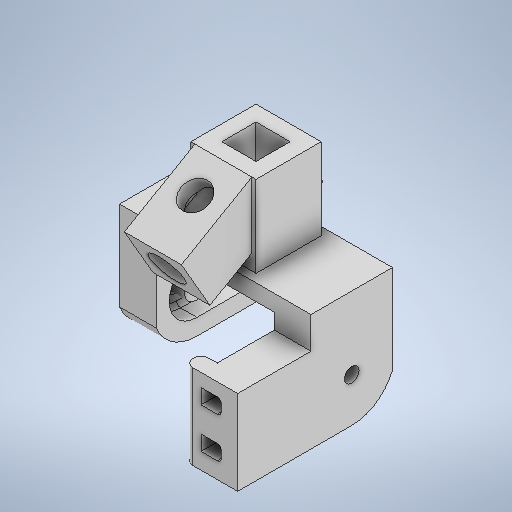
# Autodesk Inventor part: øvre del av kne Andre versjon
Saved by Autodesk Inventor 2025.1 (Build 291241020, 241B)
## iProperties
Created: 2024-10-04
Part Number: øvre del av kne Andre versjon
Material: Generic
Document SubType Name: Modeling
Designer: morte
Density: 1 g/cm^3
Appearance: Default
Author: morte
Autodesk Inventor part; units mm, degrees
ref_plane "XZ Plane" through (0, 0, 0) normal (0, 1, 0) x (-1, 0, 0)
ref_plane "XY Plane" through (0, 0, 0) normal (0, 0, 1) x (1, 0, 0)
sketch "Sketch1" plane through (0, 0, 0) normal (0, 0, 1) x (1, 0, 0)
  line L0 (0, 0) -> (0, 12.3)
  line L1 (0, 12.3) -> (14.5, 12.3)
  line L2 (14.5, 12.3) -> (14.5, 0)
  line L3 (14.5, 0) -> (19, 0)
  line L4 (19, 0) -> (19, 14.3)
  line L5 (19, 14.3) -> (-4.5, 14.3)
  line L6 (-4.5, 14.3) -> (-4.5, 0)
  line L7 (-4.5, 0) -> (0, 0)
  dimension "d6" = 12.3
  dimension "d7" = 14.5
  dimension "d8" = 4.5
  dimension "d9" = 14.3
  dimension "d10" = 23.5
  dimension "d108" = 12.3
  dimension "d205" = 4.5
  constraints: 16 end point, 3 perpendicular, 3 vertical, 2 horizontal
  measures "d6" distance of L0.start L0.end
  measures "d7" distance of L0.end L1.end
  measures "d8" distance of L2.end L3.end
  measures "d9" distance of L3.end L4.end
  measures "d10" distance of L4.end L5.end
  measures "d108" distance of L1.end L2.end
  measures "d205" distance of L6.end L0.start
extrude "Extrusion1" add sketch "Sketch1" along normal mid plane 10
sketch "Sketch2" plane through (-4.5, 14.3, 5) normal (0, 1, 0) x (1, 0, 0)
  line L0 (0, 10) -> (0, 0) projected
  line L1 (0, 10) -> (23.5, 10) projected
  line L2 (0, 0) -> (23.5, 10)
  line L3 (23.5, 0) -> (0, 0) projected
  line L4 (0, 10) -> (23.5, 0)
  line L5 (9.65, 2.9) -> (13.85, 2.9)
  line L6 (13.85, 2.9) -> (13.85, 7.1)
  line L7 (13.85, 7.1) -> (9.65, 7.1)
  line L8 (9.65, 7.1) -> (9.65, 2.9)
  line L9 (9.65, 2.9) -> (13.85, 7.1) construction
  line L10 (13.85, 2.9) -> (9.65, 7.1) construction
  line L11 (7.75, 1) -> (15.75, 1)
  line L12 (15.75, 1) -> (15.75, 9)
  line L13 (15.75, 9) -> (7.75, 9)
  line L14 (7.75, 9) -> (7.75, 1)
  line L15 (7.75, 1) -> (15.75, 9) construction
  line L16 (15.75, 1) -> (7.75, 9) construction
  point P0 (4.5, 5)
  point P1 (11.75, 5)
  dimension "d11" = 4.2
  dimension "d12" = 4.2
  dimension "d13" = 8
  dimension "d14" = 8
  constraints: 28 end point, 5 midpoint, 4 parallel, 2 horizontal, 2 perpendicular, 1 point on line
  measures "d11" distance of L6.end L7.end
  measures "d12" distance of L5.end L6.end
  measures "d13" distance of L12.end L13.end
  measures "d14" distance of L11.end L12.end
extrude "Extrusion2" add sketch "Sketch2" along normal blind 10 contours L14 L13 L12 L2 L6 L7 L8 L4 | L4 L8 L2 L14 | L2 L8 L5 L6 L4 L12 L11 L14 | L12 L4 L6 L2
sketch "Sketch3" plane through (0, 0, 5) normal (1, 0, 0) x (0, 0, -1)
  line L0 (10, 0) -> (0, 0) projected
  line L1 (0, 0) -> (5, 0)
  line L2 (10, 14.3) -> (0, 14.3) projected
  line L3 (6.95, 14.3) -> (3.05, 14.3)
  line L4 (5, 0) -> (5, 2)
  line L5 (8.4, 5.4) -> (17.767, 5.4) construction
  line L6 (6.8, 5.4) -> (16.167, 5.4) construction
  line L7 (1.6, 5.4) -> (10.967, 5.4) construction
  line L8 (3.2, 5.4) -> (12.567, 5.4) construction
  line L9 (5, 5.4) -> (5, 0)
  line L10 (5, 8.8) -> (5, 10.4)
  line L11 (5, 10.4) -> (19, 10.4)
  line L12 (5, 0) -> (19, 0)
  line L13 (19, 0) -> (19, 10.4)
  line L14 (5, 8.8) -> (5, 0)
  point P0 (1.9, 14.3)
  point P1 (8.1, 14.3)
  point P2 (10, 0)
  dimension "d17" = 5
  dimension "d111" = 2
  dimension "d172" = 1.6
  dimension "d173" = 14
  dimension "d174" = 14
  constraints: 26 end point, 6 point on line, 4 horizontal, 2 collinear, 2 perpendicular, 2 vertical, 1 midpoint
  measures "d17" distance of L0.end L1.end
  measures "d111" distance of L1.end L4.end
  measures "d172" distance of L10.start L10.end
  measures "d173" distance of L10.end L11.end
  measures "d174" distance of L12.start L12.end
extrude "Extrusion3" add sketch "Sketch3" against normal blind 4.5
ref_plane "Work Plane1" through (10.75, 0, 0) normal (1, 0, 0) x (0, 1, 0)
sketch "Sketch15" plane through (10.75, 0, 0) normal (1, 0, 0) x (0, 1, 0)
  line L0 (24.3, -4) -> (24.3, 4) projected
  line L1 (24.3, 4) -> (19.3, 12.6603)
  line L2 (24.3, 4) -> (34.3, 4) construction
  line L3 (24.3, 4) -> (16.3, 4)
  line L4 (14.3, 4) -> (24.3, 4) projected
  line L5 (19.3, 12.6603) -> (13.2378, 9.1603)
  line L6 (13.2378, 9.1603) -> (16.2171, 4)
  line L7 (13.2378, 9.1603) -> (19.1964, 9.1603) construction
  point P0 (0, 0)
  point P1 (18.5265, 4)
  dimension "d83" = 10
  dimension "d84" = 120
  dimension "d85" = 8
  dimension "d93" = 7
  dimension "d94" = 60
  constraints: 12 end point, 2 equal length, 2 horizontal, 2 point on line
  measures "d83" distance of L0.end L1.end
  measures "d84" angle of L2 L1
  measures "d85" distance of L0.end L3.end
  measures "d93" distance of L1.end L5.end
  measures "d94" angle of L6 L7
extrude "Extrusion13" add sketch "Sketch15" against normal blind 7
sketch "Sketch17" plane through (3.75, 19.3, 12.6603) normal (0, -0.5, 0.866) x (1, 0, 0)
  line L0 (7, -7) -> (0, -7) projected
  line L1 (0, 0) -> (3.5, 0)
  line L2 (3.5, 0) -> (3.5, -3.5)
  circle A0 centre (3.5, -3.5) radius 2.1
  point P0 (-3.75, -23.0444)
  point P1 (0.25, -7)
  point P2 (6.5, -7)
  dimension "d119" = 3.5
  dimension "d120" = 3.5
  dimension "d121" = 4.2
  constraints: 4 end point, 1 centre point, 1 coincident, 1 horizontal, 1 perpendicular
  measures "d119" distance of L1.start L1.end
  measures "d120" distance of L1.end L2.end
  measures "d121" diameter of A0
extrude "Extrusion15" cut sketch "Sketch17" against normal blind 13
sketch "Sketch22" plane through (14.5, 0, 5) normal (-1, 0, 0) x (0, 0, 1)
  line L0 (-10, 0) -> (0, 0) projected
  line L1 (0, 0) -> (-5, 0)
  line L2 (-5, 0) -> (0.4, 0) construction
  line L3 (9, 8.8) -> (9, 0)
  line L4 (9, 0) -> (-5, 0)
  line L5 (9, 9.4295) -> (9, 0)
  line L6 (-5, 10.4) -> (9, 10.4)
  line L7 (9, 10.4) -> (9, 9.4295)
  line L8 (-5, 10.4) -> (-5, 0)
  point P0 (0, 0)
  constraints: 16 end point, 4 collinear, 1 horizontal, 1 perpendicular
extrude "Extrusion20" add sketch "Sketch22" against normal blind 4.5
sketch "Sketch23" plane through (14.5, 0, -5) normal (-1, 0, 0) x (0, 0, 1)
  line L0 (0, 14.3) -> (0, 0) projected
  line L1 (0, 0) -> (5, 0)
  line L2 (0, 0) -> (19, 0) projected
  line L3 (5, 0) -> (5, 5.4)
  circle A0 centre (5, 5.4) radius 1.55
  circle A1 centre (5, 5.4) radius 3.4
  line L4 (5, 2) -> (20, 2)
  line L5 (5, 3.85) -> (20, 3.85)
  line L6 (5, 6.95) -> (20, 6.95)
  line L7 (5, 8.8) -> (20, 8.8)
  line L8 (20, 8.8) -> (20, 6.95)
  line L9 (20, 3.85) -> (20, 2)
  point P0 (8.0261, 3.85)
  point P1 (8.0261, 6.95)
  dimension "d161" = 5.4
  dimension "d162" = 3.1
  dimension "d163" = 6.8
  dimension "d164" = 15
  dimension "d165" = 15
  dimension "d166" = 15
  constraints: 16 end point, 4 point on circle, 4 tangent, 3 perpendicular, 2 centre point, 2 coincident, 2 horizontal, 2 point on line, 1 collinear, 1 vertical
  measures "d161" distance of L1.end L3.end
  measures "d162" diameter of A0
  measures "d163" diameter of A1
  measures "d164" distance of L4.start L4.end
  measures "d165" distance of L5.start L5.end
  measures "d166" distance of L6.start L6.end
extrude "Extrusion21" cut sketch "Sketch23" against normal blind 2.5 contours A1 L6 A0 L3 | L3 L5 A1 | A1 L5 L9 L4 | A0 L6 A1 L5 | L7 L8 L6 A1
sketch "Sketch24" plane through (14.5, 5.4, 0) normal (-1, 0, 0) x (0, 0, 1)
  circle A0 centre (0, 0) radius 0.9
  point P0 (0, -5.4)
  dimension "d169" = 1.8
  constraints: 1 centre point
  measures "d169" diameter of A0
extrude "Extrusion22" cut sketch "Sketch24" against normal through all
sketch "Sketch25" plane through (0, 0, 5) normal (1, 0, 0) x (0, 0, -1)
  line L0 (19, 0) -> (0, 0) projected
  line L1 (0, 0) -> (5, 0)
  line L2 (5, 0) -> (5, 5.4)
  line L3 (5, 0) -> (10.4, 0) construction
  circle A0 centre (5, 5.4) radius 1.55
  circle A1 centre (5, 5.4) radius 3.4
  line L4 (5, 8.8) -> (20, 8.8)
  line L5 (5, 6.95) -> (20, 6.95)
  line L6 (5, 3.85) -> (20, 3.85)
  line L7 (5, 2) -> (20, 2)
  line L8 (20, 2) -> (20, 3.85)
  line L9 (20, 6.95) -> (20, 8.8)
  point P0 (8.0261, 6.95)
  point P1 (8.0261, 3.85)
  dimension "d175" = 5.4
  dimension "d176" = 90
  dimension "d177" = 3.1
  dimension "d178" = 6.8
  dimension "d179" = 15
  dimension "d180" = 15
  dimension "d181" = 15
  dimension "d182" = 15
  constraints: 18 end point, 4 horizontal, 4 perpendicular, 4 point on circle, 4 tangent, 2 centre point, 2 coincident, 2 point on line
  measures "d175" distance of L1.end L2.end
  measures "d176" angle of L3 L2
  measures "d177" diameter of A0
  measures "d178" diameter of A1
  measures "d179" distance of L4.start L4.end
  measures "d180" distance of L5.start L5.end
  measures "d181" distance of L6.start L6.end
  measures "d182" distance of L7.start L7.end
extrude "Extrusion23" cut sketch "Sketch25" against normal blind 2.5 contours A1 L5 A0 L2 | L2 L6 A1 | A1 L6 L8 L7 | A0 L5 A1 L6 | L4 L9 L5 A1
sketch "Sketch26" plane through (0, 5.4, 0) normal (1, 0, 0) x (0, 0, -1)
  circle A0 centre (0, 0) radius 0.9
  point P0 (0, -5.4)
  dimension "d185" = 1.8
  constraints: 1 centre point
  measures "d185" diameter of A0
extrude "Extrusion24" cut sketch "Sketch26" against normal through all
sketch "Sketch27" plane through (0, 5.4, 0) normal (1, 0, 0) x (0, 0, -1)
  circle A0 centre (0, 0) radius 0.9 projected
  arc A1 (-5, -2.0396) -> (0, -5.4) centre (0, 0) ccw
  line L0 (-5, 8.9) -> (-5, -5.4) projected
  line L1 (-5, -2.0396) -> (-5, -5.4)
  line L2 (-5, -5.4) -> (0, -5.4)
  constraints: 4 end point, 3 point on circle, 2 point on line, 1 centre point, 1 coincident, 1 collinear, 1 perpendicular
extrude "Extrusion25" cut sketch "Sketch27" against normal through all contours A1 L2 L0
sketch "Sketch28" plane through (14.5, 5.4, 0) normal (-1, 0, 0) x (0, 0, 1)
  arc A0 (-5, -2.0388) -> (0.0007, -5.4) centre (0.0003, 0) ccw
  line L0 (-5, 8.9) -> (-5, -5.4) projected
  line L1 (-5, -2.0388) -> (-5, -5.4)
  line L2 (-5, -5.4) -> (0, -5.4)
  constraints: 4 end point, 3 point on circle, 2 point on line, 1 centre point, 1 collinear, 1 perpendicular
extrude "Extrusion26" cut sketch "Sketch28" against normal through all
fillet "Fillet9" radius 0.5 12 edges at (17, 8.8, 7) (17, 2, 7) (17, 5.4, -3.4) (17, 5.4, -1.55) (17, 6.95, 8.5131) (17, 3.85, 8.5131) (-2.5, 8.8, -7) (-2.5, 2, -7) (-2.5, 5.4, 3.4) (-2.5, 6.95, -8.5131) (-2.5, 3.85, -8.5131) (-2.5, 5.4, 1.55)
sketch "Sketch29" plane through (0, 3.85, -14) normal (1, 0, 0) x (0, 0, -1)
  line L0 (0, 6.55) -> (0, -3.85) projected
  line L1 (0, -3.85) -> (-2, -3.85)
  line L2 (0, -3.85) -> (-14, -3.85) projected
  line L3 (-2, -3.85) -> (-2, 6.55)
  line L4 (-9, 6.55) -> (0, 6.55) projected
  line L5 (-2, 6.55) -> (0, 6.55)
  line L6 (0, -3.85) -> (0, 6.55)
  dimension "d193" = 2
  constraints: 8 end point, 2 collinear, 2 point on line, 1 perpendicular
  measures "d193" distance of L0.end L1.end
extrude "Extrusion27" add sketch "Sketch29" along normal blind 2
sketch "Sketch30" plane through (14.5, 3.85, 14) normal (-1, 0, 0) x (0, 0, 1)
  line L0 (0, 6.55) -> (0, -3.85) projected
  line L1 (0, -3.85) -> (-2, -3.85)
  line L2 (-14, -3.85) -> (0, -3.85) projected
  line L3 (-2, -3.85) -> (-2, 6.55)
  line L4 (-9, 6.55) -> (0, 6.55) projected
  line L5 (0, 6.55) -> (0, -3.85)
  dimension "d196" = 2
  constraints: 6 end point, 2 point on line, 1 parallel, 1 perpendicular
  measures "d196" distance of L0.end L1.end
extrude "Extrusion28" add sketch "Sketch30" along normal blind 2
fillet "Fillet10" radius 1 4 edges at (12.5, 5.2, 14) (12.5, 5.2, 12) (2, 5.2, -12) (2, 5.2, -14)
sketch "Sketch31" plane through (3.75, 24.3, 4) normal (0, 0.866, 0.5) x (1, 0, 0)
  line L0 (-0.5, 0) -> (7, 0) projected
  line L1 (0, 0) -> (3.5, 0)
  line L2 (-0.5, 0) -> (7.5, 0) projected
  line L3 (3.5, 0) -> (3.5, -4)
  circle A0 centre (3.5, -4) radius 1.75
  point P0 (-3.75, -8.6859)
  dimension "d200" = 3.5
  dimension "d201" = 4
  dimension "d202" = 3.5
  constraints: 4 end point, 1 centre point, 1 coincident, 1 midpoint, 1 perpendicular
  measures "d200" distance of L1.start L1.end
  measures "d201" distance of L1.end L3.end
  measures "d202" diameter of A0
extrude "Extrusion29" cut sketch "Sketch31" against normal blind 2
body "Solid1"
